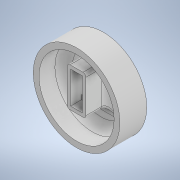
# Autodesk Inventor part: podstawa 01-4
Saved by Autodesk Inventor 2021 (Build 250183000, 183)
## iProperties
Created: 2022-02-04
Part Number: podstawa 01-4
Material: Generic
Document SubType Name: Modeling
Designer: Łukasz
Density: 1 g/cm^3
Appearance: Default
Author: Łukasz
Autodesk Inventor part; units mm, degrees
ref_plane "YZ Plane" through (0, 0, 0) normal (1, 0, 0) x (0, 1, 0)
ref_plane "XZ Plane" through (0, 0, 0) normal (0, 1, 0) x (-1, 0, 0)
ref_plane "XY Plane" through (0, 0, 0) normal (0, 0, 1) x (1, 0, 0)
sketch "Sketch1" plane through (0, 0, 0) normal (0, 0, 1) x (1, 0, 0)
  circle A0 centre (0, 0) radius 75
  dimension "d0" = 150
  constraints: 1 centre point, 1 coincident
  measures "d0" diameter of A0
extrude "Extrusion1" add sketch "Sketch1" along normal blind 46.5
sketch "Sketch2" plane through (0, 0, 46.5) normal (0, 0, 1) x (1, 0, 0)
  line L0 (-10.25, 30.375) -> (10.25, 30.375)
  line L1 (10.25, 30.375) -> (10.25, -10.125)
  line L2 (10.25, -10.125) -> (-10.25, -10.125)
  line L3 (-10.25, -10.125) -> (-10.25, 30.375)
  line L4 (3.25, -10.125) -> (-3.25, -10.125)
  line L5 (-3.25, -10.125) -> (-3.25, -15.125)
  line L6 (-3.25, -15.125) -> (3.25, -15.125)
  line L7 (3.25, -15.125) -> (3.25, -10.125)
  point P0 (0, 0)
  point P1 (-3.25, -10.125)
  dimension "d5" = 20.5
  dimension "d6" = 40.5
  dimension "d8" = 10.125
  dimension "d9" = 10.25
  dimension "d10" = 6.5
  dimension "d11" = 5
  dimension "d12" = 0
  dimension "d13" = 7
  constraints: 16 end point, 4 parallel, 2 horizontal, 2 perpendicular, 1 other
  measures "d5" distance of L1.end L2.end
  measures "d6" distance of L0.end L1.end
  measures "d8" distance from line of point (0, 0) L2
  measures "d9" distance from line of point (0, 0) L3
  measures "d10" distance of L6.end L5.end
  measures "d11" distance of L5.end L4.end
  measures "d12" distance between parallel lines of L2 L4
  measures "d13" distance between parallel lines of L3 L5
extrude "Extrusion2" cut sketch "Sketch2" against normal up to surface (46.5 mm away)
sketch "Sketch4" plane through (0, 0, 0) normal (0, 0, -1) x (-1, 0, 0)
  line L0 (2.5, -79.3047) -> (-2.5, -79.3047)
  line L1 (-2.5, -79.3047) -> (-2.5, -3.4585)
  line L2 (-2.5, -3.4585) -> (2.5, -3.4585)
  line L3 (2.5, -3.4585) -> (2.5, -79.3047)
  line L4 (-3.25, -15.125) -> (-3.25, -10.125) projected
  point P0 (0, 0)
  dimension "d16" = 5
  dimension "d17" = 0.75
  constraints: 8 end point, 2 parallel, 1 horizontal, 1 perpendicular
  measures "d16" distance of L1.end L2.end
  measures "d17" distance between parallel lines of L4 L1
extrude "Extrusion3" cut sketch "Sketch4" against normal blind 2.5
sketch "Sketch5" plane through (0, 0, 46.5) normal (0, 0, 1) x (1, 0, 0)
  line L0 (10.25, -17.625) -> (-10.25, -17.625)
  line L1 (-10.25, -17.625) -> (-10.25, 37.875)
  line L2 (-10.25, 37.875) -> (10.25, 37.875)
  line L3 (10.25, 37.875) -> (10.25, -17.625)
  line L4 (-10.25, 30.375) -> (10.25, 30.375) projected
  point P0 (0, 0)
  dimension "d20" = 55.5
  dimension "d21" = 7.5
  constraints: 8 end point, 2 parallel, 1 horizontal, 1 perpendicular
  measures "d20" distance of L0.end L1.end
  measures "d21" distance between parallel lines of L4 L2
extrude "Extrusion4" cut sketch "Sketch5" against normal blind 19
sketch "Sketch6" plane through (0, 0, 46.5) normal (0, 0, 1) x (1, 0, 0)
  circle A0 centre (0, 0) radius 75 projected
  circle A1 centre (0, 0) radius 65
  line L0 (-10.25, -17.625) -> (-10.25, 37.875) projected
  line L1 (-10.25, 37.875) -> (10.25, 37.875) projected
  line L2 (10.25, 37.875) -> (10.25, -17.625) projected
  line L3 (10.25, -17.625) -> (-10.25, -17.625) projected
  line L4 (16.25, 43.875) -> (-16.25, 43.875)
  line L5 (-16.25, 43.875) -> (-16.25, -23.625)
  line L6 (-16.25, -23.625) -> (16.25, -23.625)
  line L7 (16.25, -23.625) -> (16.25, 43.875)
  dimension "d24" = 10
  dimension "d25" = 6
  constraints: 8 end point, 1 centre point, 3 other
  measures "d24" radial gap between concentric circles of A0 A1
  measures "d25" distance between parallel lines of L1 L4
extrude "Extrusion5" cut sketch "Sketch6" against normal blind 42.5 contours A1
fillet "Fillet1" radius 15 5 edges at (-16.25, 10.125, 4) (0, 43.875, 4) (16.25, 10.125, 4) (0, -23.625, 4) (-65, 0, 4)
fillet "Fillet2" radius 5 11 edges at (-20.6434, -28.0184, 8.3934) (-16.25, -23.625, 32.75) (20.6434, -28.0184, 8.3934) (16.25, -23.625, 32.75) (-16.25, 10.125, 19) (0, 43.875, 19) (-18.3718, 45.9968, 11.3089) (-16.25, 43.875, 32.75) (16.25, 10.125, 19) (18.3718, 45.9968, 11.3089) (16.25, 43.875, 32.75)
sketch "Sketch7" plane through (0, 0, 4) normal (0, 0, 1) x (1, 0, 0)
  line L0 (0, 0) -> (-35.3553, 35.3553) construction
  arc A0 (-31.25, 39.0312) -> (31.25, 39.0312) centre (0, 0) ccw projected
  line L1 (0, 0) -> (50, 0) construction
  circle A1 centre (-35.3553, 35.3553) radius 2
  line L2 (0, 0) -> (-35.3553, -35.3553) construction
  circle A2 centre (-35.3553, -35.3553) radius 2
  line L3 (0, 0) -> (35.3553, -35.3553) construction
  circle A3 centre (35.3553, -35.3553) radius 2
  line L4 (0, 0) -> (35.3553, 35.3553) construction
  circle A4 centre (35.3553, 35.3553) radius 2
  dimension "d30" = 135
  dimension "d31" = 4
  dimension "d34" = 360
  constraints: 10 end point, 6 coincident, 4 centre point, 1 equal length, 1 horizontal, 1 point on circle, 19 other
  measures "d30" angle of L1 L0
  measures "d31" diameter of A1
extrude "Extrusion6" cut sketch "Sketch7" along normal blind 41.5 and the other way blind 20.75
sketch "Sketch8" plane through (0, 0, 4) normal (0, 0, 1) x (1, 0, 0)
  arc A0 (-36.741, 33.9131) -> (-33.9131, 36.741) centre (-35.3553, 35.3553) ccw projected
  circle A1 centre (-35.3553, 35.3553) radius 5
  circle A2 centre (-35.3553, -35.3553) radius 5
  circle A3 centre (35.3553, -35.3553) radius 5
  circle A4 centre (35.3553, 35.3553) radius 5
  point P0 (0, 0)
  dimension "d40" = 10
  dimension "d43" = 360
  constraints: 4 centre point, 1 coincident, 9 other
  measures "d40" diameter of A1
extrude "Extrusion7" cut sketch "Sketch8" along normal blind 41.5
equation "\"d9\" = 0.5 * d5"
equation "\"d13\" = 0.5 * d5 - 0.5 * d10"
body "Solid1"
